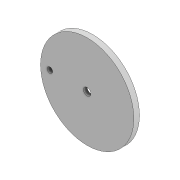
# Autodesk Inventor part: rueda
Saved by Autodesk Inventor 2022 (Build 260153000, 153)
## iProperties
Created: 2022-11-06
Part Number: rueda
Material: Genérico
Document SubType Name: Modeling
Designer: Jorge
Density: 1 g/cm^3
Appearance: Valor por defecto
Author: Jorge
Autodesk Inventor part; units mm, degrees
ref_plane "YZ Plane" through (0, 0, 0) normal (1, 0, 0) x (0, 1, 0)
ref_plane "XZ Plane" through (0, 0, 0) normal (0, 1, 0) x (-1, 0, 0)
ref_plane "XY Plane" through (0, 0, 0) normal (0, 0, 1) x (1, 0, 0)
sketch "Boceto1" plane through (0, 0, 0) normal (0, 0, 1) x (1, 0, 0)
  circle A0 centre (0, 0) radius 25
  dimension "d0" = 50
  constraints: 1 centre point, 1 coincident
  measures "d0" diameter of A0
extrude "Extrusión1" add sketch "Boceto1" along normal blind 3
sketch "Boceto2" plane through (0, 0, 3) normal (0, 0, 1) x (1, 0, 0)
  circle A0 centre (0, 0) radius 2
  dimension "d3" = 4
  constraints: 1 centre point, 1 coincident
  measures "d3" diameter of A0
extrude "Extrusión2" cut sketch "Boceto2" against normal blind 3
sketch "Boceto3" plane through (0, 0, 3) normal (0, 0, 1) x (1, 0, 0)
  circle A0 centre (0, 0) radius 2 construction
  circle A1 centre (0, 0) radius 25 construction
  line L0 (0, 0) -> (-25, 0) construction
  circle A2 centre (0, 0) radius 25 construction
  circle A3 centre (-20, 0) radius 1.5
  dimension "d6" = 3
  dimension "d7" = 20
  constraints: 2 end point, 1 centre point, 1 horizontal, 1 horizontal alignment, 1 point on line, 1 other
  measures "d6" diameter of A3
  measures "d7" distance of point (0, 0) A3.centre
extrude "Extrusión3" cut sketch "Boceto3" against normal blind 3
sketch "Boceto4" plane through (0, 0, 0) normal (0, 0, -1) x (-1, 0, 0)
  arc A0 (-17.5, -1.5) -> (-15.5, -3.5) centre (-15.5, -1.5) ccw construction
  line L0 (-2, -3.5) -> (-15.5, -3.5) construction
  line L1 (-2, -6.5) -> (-2, -3.5) construction
  arc A1 (-2, -6.5) -> (2, -6.5) centre (0, -6.5) ccw construction
  line L2 (2, -3.5) -> (2, -6.5) construction
  line L3 (15.5, -3.5) -> (2, -3.5) construction
  arc A2 (15.5, -3.5) -> (17.5, -1.5) centre (15.5, -1.5) ccw construction
  line L4 (17.5, 1.5) -> (17.5, -1.5) construction
  arc A3 (17.5, 1.5) -> (15.5, 3.5) centre (15.5, 1.5) ccw construction
  line L5 (2, 3.5) -> (15.5, 3.5) construction
  line L6 (2, 6.5) -> (2, 3.5) construction
  arc A4 (2, 6.5) -> (-2, 6.5) centre (0, 6.5) ccw construction
  line L7 (-2, 3.5) -> (-2, 6.5) construction
  line L8 (-15.5, 3.5) -> (-2, 3.5) construction
  arc A5 (-15.5, 3.5) -> (-17.5, 1.5) centre (-15.5, 1.5) ccw construction
  line L9 (-17.5, -1.5) -> (-17.5, 1.5) construction
  line L10 (0, 8.5) -> (0, -8.5) construction
  line L11 (-17.5, 0) -> (17.5, 0) construction
  line L12 (-2.25, 3.75) -> (-2.25, 6.5)
  arc A6 (2.25, 6.5) -> (-2.25, 6.5) centre (0, 6.5) ccw
  line L13 (2.25, 6.5) -> (2.25, 3.75)
  line L14 (2.25, 3.75) -> (15.5, 3.75)
  arc A7 (17.75, 1.5) -> (15.5, 3.75) centre (15.5, 1.5) ccw
  line L15 (17.75, 1.5) -> (17.75, -1.5)
  arc A8 (15.5, -3.75) -> (17.75, -1.5) centre (15.5, -1.5) ccw
  line L16 (15.5, -3.75) -> (2.25, -3.75)
  line L17 (2.25, -3.75) -> (2.25, -6.5)
  arc A9 (-2.25, -6.5) -> (2.25, -6.5) centre (0, -6.5) ccw
  line L18 (-2.25, -6.5) -> (-2.25, -3.75)
  line L19 (-2.25, -3.75) -> (-15.5, -3.75)
  arc A10 (-17.75, -1.5) -> (-15.5, -3.75) centre (-15.5, -1.5) ccw
  line L20 (-17.75, -1.5) -> (-17.75, 1.5)
  arc A11 (-15.5, 3.75) -> (-17.75, 1.5) centre (-15.5, 1.5) ccw
  line L21 (-15.5, 3.75) -> (-2.25, 3.75)
  point P0 (0, 0)
  point P1 (17.5, -3.5)
  point P2 (0, 0)
  dimension "d10" = 0.25
  constraints: 44 end point, 26 point on circle, 12 centre point, 3 midpoint, 15 other
  measures "d10" distance between parallel lines of L8 L21
extrude "Extrusión4" cut sketch "Boceto4" against normal blind 1
